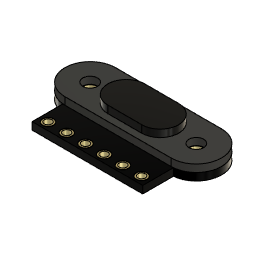
TOF200C (Autodesk Fusion 360 design; units mm, degrees)
Autodesk Fusion 360 part; units mm, degrees
sketch "Sketch1" plane through (0, 0, 0) normal (0, 0, 1) x (1, 0, 0) in component "PCB"
  line L0 (-7.2, -3.425) -> (7.2, -3.425)
  arc A0 (7.2, -3.425) -> (7.2, 3.425) centre (7.2, 0) ccw
  line L1 (7.2, 3.425) -> (-7.2, 3.425)
  arc A1 (-7.2, 3.425) -> (-7.2, -3.425) centre (-7.2, 0) ccw
  line L2 (-7.2, 0) -> (7.2, 0) construction
  circle A2 centre (-7.2, 0) radius 1
  circle A3 centre (7.2, 0) radius 1
  line L3 (-7.5, -7.575) -> (7.5, -7.575)
  line L4 (-7.5, -7.575) -> (-7.5, -3.4118)
  line L5 (7.5, -7.575) -> (7.5, -3.4118)
  circle A4 centre (-6.35, -6.575) radius 0.5
  circle A5 centre (-3.81, -6.575) radius 0.5
  circle A6 centre (-1.27, -6.575) radius 0.5
  circle A7 centre (1.27, -6.575) radius 0.5
  circle A8 centre (3.81, -6.575) radius 0.5
  circle A9 centre (6.35, -6.575) radius 0.5
  circle A10 centre (-6.35, -6.575) radius 0.75
  circle A11 centre (-3.81, -6.575) radius 0.75
  circle A12 centre (-1.27, -6.575) radius 0.75
  circle A13 centre (1.27, -6.575) radius 0.75
  circle A14 centre (3.81, -6.575) radius 0.75
  circle A15 centre (6.35, -6.575) radius 0.75
  circle A16 centre (-7.2, 0) radius 1.5
  circle A17 centre (7.2, 0) radius 1.5
  dimension "d1" = 6.85
  dimension "d2" = 14.4
  dimension "d3" = 2
  dimension "d4" = 2
  dimension "d5" = 11
  dimension "d6" = 15
  dimension "d7" = 7.5
  dimension "d8" = 1
  dimension "d11" = 2.54
  dimension "d12" = 0
  dimension "d13" = 1.27
  dimension "d14" = 1
  dimension "d15" = 1.5
  dimension "d16" = 3
  dimension "d17" = 3
  constraint tangent L0 A0
  constraint tangent A0 L1
  constraint parallel L0 L1
  constraint tangent L1 A1
  constraint tangent L0 A1
  constraint horizontal L2
  constraint midpoint L2 origin
  constraint concentric A1 A2
  constraint concentric A0 A3
  constraint horizontal L3
  constraint coincident A1 L4.end
  constraint perpendicular L3 L4
  constraint coincident A0 L5.end
  constraint perpendicular L3 L5
  constraint concentric A4 A10
  constraint concentric A1 A16
  constraint concentric A0 A17
  measures "d1" diameter of A0
  measures "d2" distance of A1.centre A0.centre
  measures "d3" diameter of A2
  measures "d4" diameter of A3
  measures "d5" distance of L1 L3
  measures "d6" distance of L3.start L3.end
  measures "d7" horizontal distance of origin L3.end
  measures "d8" diameter of A4
  measures "d13" horizontal distance of origin A6.centre
  measures "d14" distance of L3 A4.centre
  measures "d15" diameter of A10
  measures "d16" diameter of A16
  measures "d17" diameter of A17
extrude "Extrude1" add sketch "Sketch1" against normal blind 1 contours L0 A0 L1 A1 | L0 A0 A1 L3 L4 L5 | A10 | A11 | A12 | A13 | A14 | A15 | A16 | A17 makes body 1 in component "PCB"
extrude "Extrude2" add sketch "Sketch1" along normal blind 0.05 contours A10 | A11 | A12 | A13 | A14 | A15 | A16 | A17 bodies 1 in component "PCB"
extrude "Extrude3" add 8 faces at (-5.8723, -0.0745, 0.05) (8.524, -0.1242, 0.05) (7.0139, -6.6123, 0.05) (4.472, -6.6371, 0.05) (1.932, -6.6371, 0.05) (-0.608, -6.6371, 0.05) (-3.1461, -6.6123, 0.05) (-5.6861, -6.6123, 0.05) along direction (0, 0, -1) blind 0.05 start surface through (0, 0, -1) normal (0, 0, -1) on bodies 1 bodies 1 in component "PCB"
sketch "Sketch1 (2)" plane through (0, 0, 0) normal (0, 0, 1) x (1, 0, 0) in component "Lens"
  line L0 (7.2, 3.425) -> (-7.2, 3.425)
  arc A0 (-7.2, 3.425) -> (-7.2, -3.425) centre (-7.2, 0) ccw
  arc A1 (7.2, -3.425) -> (7.2, 3.425) centre (7.2, 0) ccw
  line L1 (-7.2, -3.425) -> (7.2, -3.425)
  line L2 (-2.3, -2.5) -> (2.3, -2.5)
  arc A2 (2.3, -2.5) -> (2.3, 2.5) centre (2.3, 0) ccw
  line L3 (2.3, 2.5) -> (-2.3, 2.5)
  arc A3 (-2.3, 2.5) -> (-2.3, -2.5) centre (-2.3, 0) ccw
  line L4 (-2.3, 0) -> (2.3, 0) construction
  circle A4 centre (-7.2, 0) radius 1
  circle A5 centre (7.2, 0) radius 1
  dimension "d25" = 5
  dimension "d26" = 4.6
  constraint tangent L2 A2
  constraint tangent A2 L3
  constraint parallel L2 L3
  constraint tangent L3 A3
  constraint tangent L2 A3
  constraint horizontal L4
  constraint midpoint L4 origin
  measures "d25" diameter of A2
  measures "d26" distance of A3.centre A2.centre
extrude "Extrude1'" add sketch "Sketch1 (2)" along normal blind 1 separate body makes body 2 in component "Lens"
extrude "Extrude2'" add sketch "Sketch1 (2)" along normal blind 2 separate body contours L2 A2 L3 A3 makes body 3 in component "Lens"
sketch "Sketch1 (3)" plane through (0, 0, -1) normal (0, 0, -1) x (1, 0, 0) in component "Components"
  circle A0 centre (-6.35, 6.575) radius 0.75
  circle A1 centre (-1.27, 6.575) radius 0.75
  circle A2 centre (3.81, 6.575) radius 0.75
  circle A3 centre (7.2, 0) radius 1.5
  circle A4 centre (-7.2, 0) radius 1.5
  circle A5 centre (6.35, 6.575) radius 0.75
  circle A6 centre (1.27, 6.575) radius 0.75
  circle A7 centre (-3.81, 6.575) radius 0.75
  line L0 (7.5, 7.575) -> (-7.5, 7.575)
  line L1 (-7.5, 7.575) -> (-7.5, 3.4118)
  arc A8 (-7.5, 3.4118) -> (-7.2, -3.425) centre (-7.2, 0) ccw
  line L2 (-7.2, -3.425) -> (7.2, -3.425)
  arc A9 (7.2, -3.425) -> (7.5, 3.4118) centre (7.2, 0) ccw
  line L3 (7.5, 3.4118) -> (7.5, 7.575)
  line L4 (4.7838, -0.6803) -> (1.8624, -0.6803)
  line L5 (1.8624, -0.6803) -> (1.8624, 0.8078)
  line L6 (1.8624, 0.8078) -> (4.7838, 0.8078)
  line L7 (4.7838, 0.8078) -> (4.7838, -0.6803)
  line L8 (1.2338, -2.372) -> (0.3043, -2.372)
  line L9 (0.3043, -2.372) -> (0.3043, -0.6868)
  line L10 (0.3043, -0.6868) -> (1.2338, -0.6868)
  line L11 (1.2338, -0.6868) -> (1.2338, -2.372)
  line L12 (1.2472, 0.8645) -> (0.341, 0.8645)
  line L13 (0.341, 0.8645) -> (0.341, 2.5965)
  line L14 (0.341, 2.5965) -> (1.2472, 2.5965)
  line L15 (1.2472, 2.5965) -> (1.2472, 0.8645)
  line L16 (-0.3513, -0.2126) -> (-2.2662, -0.2126)
  line L17 (-2.2662, -0.2126) -> (-2.2662, -1.7212)
  line L18 (-2.2662, -1.7212) -> (-0.3513, -1.7212)
  line L19 (-0.3513, -1.7212) -> (-0.3513, -0.2126)
  line L20 (-0.4521, 2.7987) -> (-2.3346, 2.7987)
  line L21 (-2.3346, 2.7987) -> (-2.3346, 1.8507)
  line L22 (-2.3346, 1.8507) -> (-0.4521, 1.8507)
  line L23 (-0.4521, 1.8507) -> (-0.4521, 2.7987)
  line L24 (-3.1873, 1.8629) -> (-4.3, 1.8629)
  line L25 (-4.3, 1.8629) -> (-4.3, 2.4)
  line L26 (-4.3, 2.4) -> (-3.1873, 2.4)
  line L27 (-3.1873, 2.4) -> (-3.1873, 1.8629)
  line L28 (-3.1785, 1) -> (-4.3, 1)
  line L29 (-4.3, 1) -> (-4.3, 0.4629)
  line L30 (-4.3, 0.4629) -> (-3.1785, 0.4629)
  line L31 (-3.1785, 0.4629) -> (-3.1785, 1)
  line L32 (-3.2, -2.4) -> (-5.2, -2.4)
  line L33 (-5.2, -2.4) -> (-5.2, -1.5)
  line L34 (-5.2, -1.5) -> (-3.2, -1.5)
  line L35 (-3.2, -1.5) -> (-3.2, -2.4)
  constraint horizontal L4
  constraint vertical L5
  constraint horizontal L6
  constraint vertical L7
  constraint horizontal L8
  constraint vertical L9
  constraint horizontal L10
  constraint vertical L11
  constraint horizontal L12
  constraint vertical L13
  constraint horizontal L14
  constraint vertical L15
  constraint horizontal L16
  constraint vertical L17
  constraint horizontal L18
  constraint vertical L19
  constraint horizontal L20
  constraint vertical L21
  constraint horizontal L22
  constraint vertical L23
  constraint horizontal L24
  constraint vertical L25
  constraint horizontal L26
  constraint vertical L27
  constraint horizontal L28
  constraint vertical L29
  constraint horizontal L30
  constraint vertical L31
  constraint horizontal L32
  constraint vertical L33
  constraint horizontal L34
  constraint vertical L35
extrude "Extrude1''" add sketch "Sketch1 (3)" along normal blind 0.5 separate body contours L4 L5 L6 L7 | L8 L9 L10 L11 | L12 L13 L14 L15 | L16 L17 L18 L19 | L20 L21 L22 L23 makes body 4 at (0.924, 1.8103, -1) makes body 5 at (-1.6279, 0.7155, -1) makes body 6 at (0.6431, -2.0192, -1) makes body 7 at (3.81, 0.1843, -1) makes body 8 at (-1.0796, -2.1667, -1) in component "Components"
extrude "Extrude2''" add sketch "Sketch1 (3)" along normal blind 0.3 separate body contours L24 L25 L26 L27 | L28 L29 L30 L31 | L32 L33 L34 L35 makes body 9 at (-3.8667, 2.1, -1) makes body 10 at (-3.9262, -0.821, -1) makes body 11 at (-3.5582, -2.0419, -1) in component "Components"
component "PCB" placed x (1, 0, 0) y (0, 1, 0) z (0, 0, 1) at (0, 0, 0)
component "Lens" placed x (1, 0, 0) y (0, 1, 0) z (0, 0, 1) at (0, 0, 0)
component "Components" placed x (1, 0, 0) y (0, 1, 0) z (0, 0, 1) at (0, 0, 0)
equation "d7 = d6 / 2"
equation "d26 = 9.6 mm - 5 mm"
